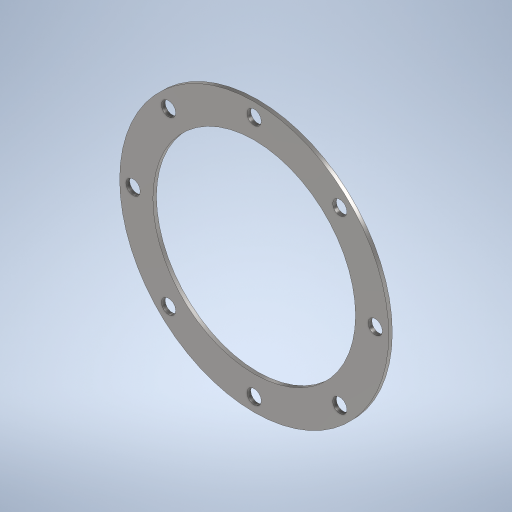
# Autodesk Inventor part: stainless steel end
Saved by Autodesk Inventor 2023 (Build 270158000, 158)
## iProperties
Created: 2022-09-19
Part Number: stainless steel end
Material: Stainless Steel
Document SubType Name: Modeling
Designer: station
Density: 8 g/cm^3
Appearance: Semi-Polished
Author: station
Autodesk Inventor part; units mm, degrees
ref_plane "YZ Plane" through (0, 0, 0) normal (1, 0, 0) x (0, 1, 0)
ref_plane "XZ Plane" through (0, 0, 0) normal (0, 1, 0) x (-1, 0, 0)
ref_plane "XY Plane" through (0, 0, 0) normal (0, 0, 1) x (1, 0, 0)
sketch "Sketch1" plane through (0, 0, 0) normal (0, 0, 1) x (1, 0, 0)
  circle A0 centre (0, 0) radius 56.5
  circle A1 centre (0, 0) radius 75
  circle A2 centre (0, 0) radius 67.5
  circle A3 centre (0, 67.5) radius 4
  circle A4 centre (47.7297, 47.7297) radius 4
  circle A5 centre (67.5, 0) radius 4
  circle A6 centre (47.7297, -47.7297) radius 4
  circle A7 centre (0, -67.5) radius 4
  circle A8 centre (-47.7297, -47.7297) radius 4
  circle A9 centre (-67.5, 0) radius 4
  circle A10 centre (-47.7297, 47.7297) radius 4
  circle A11 centre (0, 0) radius 59.5
  circle A12 centre (0, 0) radius 61.5
  dimension "d4" = 135
  dimension "d0" = 113
  dimension "d1" = 150
  dimension "d5" = 8
  dimension "d8" = 360
  dimension "d17" = 119
  dimension "d18" = 123
  constraints: 12 centre point, 7 coincident, 1 vertical alignment, 25 other
  measures "d0" diameter of A0
  measures "d1" diameter of A1
  measures "d5" diameter of A3
  measures "d17" diameter of A11
  measures "d18" diameter of A12
extrude "Extrusion1" add sketch "Sketch1" along normal blind 2 contours A1 | A2 A5 | A2 A5 | A5 A2 A6 A7 A8 A9 A10 A3 A4 | A4 A2 | A2 A4 | A6 A2 | A2 A6 | A3 A2 | A2 A3 | A7 A2 | A2 A7 | A10 A2 | A2 A10 | A8 A2 | A2 A8 | A9 A2 | A2 A9 | A11 | A12
hole "Hole2" at (0, 67.5, 0) at (47.7297, 47.7297, 0) at (67.5, 0, 0) at (47.7297, -47.7297, 0) at (0, -67.5, 0) at (-47.7297, -47.7297, 0) at (-67.5, 0, 0) at (-47.7297, 47.7297, 0) direction (0, 0, 1) diameter 8 end through all
body "Solid1"
